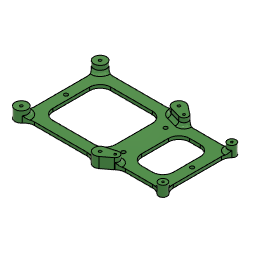
RFVplotter-PiAndMotorDriverMountingBracket-v1_0 (Autodesk Fusion 360 design; units mm, degrees)
Autodesk Fusion 360 part; units mm, degrees
sketch "Sketch1" plane through (0, 0, 0) normal (0, 1, 0) x (1, 0, 0)
  line L0 (72.5, 45) -> (-72.5, 45)
  line L1 (-72.5, 45) -> (-72.5, -45)
  line L2 (-72.5, -45) -> (72.5, -45)
  line L3 (72.5, -45) -> (72.5, 45)
  line L4 (72.5, 45) -> (-72.5, -45) construction
  line L5 (-72.5, 45) -> (72.5, -45) construction
  dimension "d1" = 90
  dimension "d2" = 145
  constraint horizontal L0
  constraint perpendicular L0 L1
  constraint parallel L0 L2
  constraint parallel L1 L3
  constraint coincident L4 origin
  constraint coincident L5 origin
  measures "d1" distance of L0.end L1.end
  measures "d2" distance of L1.end L2.end
extrude "Extrude1" add sketch "Sketch1" along normal blind 3 contours L0 L1 L2 L3 picked at (-24.166667, -15)
sketch "Sketch2" plane through (0, 3, 0) normal (0, 1, 0) x (-1, 0, 0)
  line L0 (-72.5, 45) -> (-72.5, -45)
  line L1 (-72.5, -45) -> (72.5, -45)
  line L2 (72.5, -45) -> (72.5, 45)
  line L3 (72.5, 45) -> (-72.5, 45)
  line L4 (65, -37.5) -> (-10, -37.5) construction
  line L5 (-10, -37.5) -> (-10, 37.5) construction
  line L6 (-10, 37.5) -> (65, 37.5) construction
  line L7 (65, 37.5) -> (65, -37.5) construction
  line L8 (65, -37.5) -> (-10, 37.5) construction
  line L9 (-10, -37.5) -> (65, 37.5) construction
  line L10 (0, 0) -> (72.5, 0) construction
  circle A0 centre (65, -37.5) radius 2.25 construction
  point P0 (27.5, 0)
  point P1 (65, 37.5)
  point P2 (-10, 37.5)
  point P3 (-10, -37.5)
  dimension "d5" = 75
  dimension "d6" = 75
  dimension "d7" = 4.5
  dimension "d8" = 7.5
  constraint horizontal L4
  constraint perpendicular L4 L5
  constraint parallel L4 L6
  constraint parallel L5 L7
  constraint coincident L8 P0
  constraint coincident L9 P0
  constraint midpoint L8 P0
  constraint coincident L10.start origin
  constraint midpoint L2 L10.end
  constraint coincident P0 L10
  constraint coincident L4.start L7.end
  constraint coincident P1 L6.end
  constraint coincident P2 L5.end
  constraint coincident P3 L4.end
  measures "d5" distance of L4 L6
  measures "d6" distance of P2 P1
  measures "d7" diameter of A0
  measures "d8" distance of L2 L7
hole "Hole1" at (-65, 3, 37.5) at (-65, 3, -37.5) at (10, 3, 37.5) at (10, 3, -37.5) direction (0, -1, 0) diameter 2.5 end through all
sketch "Sketch3" plane through (0, 3, 0) normal (0, 1, 0) x (-1, 0, 0)
  circle A0 centre (-10, 37.5) radius 1.25
  circle A1 centre (65, 37.5) radius 1.25
  circle A2 centre (65, -37.5) radius 1.25
  circle A3 centre (-10, -37.5) radius 1.25
  line L0 (-72.5, 45) -> (-72.5, -45)
  line L1 (-72.5, -45) -> (72.5, -45)
  line L2 (72.5, -45) -> (72.5, 45)
  line L3 (72.5, 45) -> (-72.5, 45)
  line L4 (-19.5, -32.75) -> (-65, -32.75) construction
  line L5 (-65, -32.75) -> (-65, 32.75) construction
  line L6 (-65, 32.75) -> (-19.5, 32.75) construction
  line L7 (-19.5, 32.75) -> (-19.5, -32.75) construction
  line L8 (-19.5, -32.75) -> (-65, 32.75) construction
  line L9 (-65, -32.75) -> (-19.5, 32.75) construction
  line L10 (0, 0) -> (-8.486168, 0)
  line L11 (-8.486168, 0) -> (-72.5, 0) construction
  point P0 (-42.25, 0)
  point P1 (-19.5, -32.75)
  point P2 (-65, -32.75)
  point P3 (-65, 32.75)
  point P4 (-19.5, 32.75)
  dimension "d12" = 65.5
  dimension "d13" = 45.5
  dimension "d14" = 7.5
  constraint horizontal L4
  constraint perpendicular L4 L5
  constraint parallel L4 L6
  constraint parallel L5 L7
  constraint coincident L8 P0
  constraint coincident L9 P0
  constraint coincident L10.start origin
  constraint perpendicular L7 L10
  constraint midpoint L0 L11.end
  constraint coincident P0 L11
  constraint coincident P1 L4.start
  constraint coincident P2 L4.end
  constraint coincident P3 L5.end
  constraint coincident P4 L6.end
  measures "d12" distance of P2 P3
  measures "d13" distance of P3 P4
  measures "d14" distance of L0 L5
hole "Hole2" at (19.5, 3, -32.75) at (65, 3, -32.75) at (65, 3, 32.75) at (19.5, 3, 32.75) direction (0, -1, 0) diameter 2 end through all
sketch "Sketch4" plane through (0, 3, 0) normal (0, 1, 0) x (-1, 0, 0)
  circle A0 centre (-65, 32.75) radius 1
  circle A1 centre (-19.5, -32.75) radius 1
  circle A2 centre (-65, -32.75) radius 1
  circle A3 centre (-19.5, 32.75) radius 1
  circle A4 centre (-10, 37.5) radius 1.25
  circle A5 centre (65, 37.5) radius 1.25
  circle A6 centre (65, -37.5) radius 1.25
  circle A7 centre (-10, -37.5) radius 1.25
  line L0 (-72.5, 45) -> (-72.5, -45)
  line L1 (-72.5, -45) -> (72.5, -45)
  line L2 (72.5, -45) -> (72.5, 45)
  line L3 (72.5, 45) -> (-72.5, 45)
  circle A8 centre (65, -37.5) radius 6
  circle A9 centre (65, 37.5) radius 6
  circle A10 centre (-10, -37.5) radius 6
  circle A11 centre (-10, 37.5) radius 6
  circle A12 centre (-19.5, -32.75) radius 4
  circle A13 centre (-65, -32.75) radius 4
  circle A14 centre (-19.5, 32.75) radius 4
  circle A15 centre (-65, 32.75) radius 4
  line L4 (65, -37.5) -> (-10, -37.5)
  line L5 (-10, -37.5) -> (-10, 37.5)
  line L6 (-10, 37.5) -> (65, 37.5)
  line L7 (65, 37.5) -> (65, -37.5)
  line L8 (65, -37.5) -> (-10, 37.5) construction
  line L9 (-10, -37.5) -> (65, 37.5) construction
  line L10 (-19.5, -32.75) -> (-65, -32.75)
  line L11 (-65, -32.75) -> (-65, 32.75)
  line L12 (-65, 32.75) -> (-19.5, 32.75)
  line L13 (-19.5, 32.75) -> (-19.5, -32.75)
  line L14 (-19.5, -32.75) -> (-65, 32.75) construction
  line L15 (-65, -32.75) -> (-19.5, 32.75) construction
  line L16 (-13.645808, -42.2653) -> (-21.930539, -35.926867)
  line L17 (-21.930539, 35.926867) -> (-13.645808, 42.2653)
  point P0 (27.5, 0)
  point P1 (-42.25, 0)
  dimension "d18" = 12
  dimension "d19" = 12
  dimension "d20" = 12
  dimension "d21" = 12
  dimension "d22" = 8
  dimension "d23" = 8
  dimension "d24" = 8
  dimension "d25" = 8
  constraint concentric A6 A8
  constraint concentric A5 A9
  constraint concentric A7 A10
  constraint concentric A4 A11
  constraint concentric A1 A12
  constraint concentric A2 A13
  constraint concentric A3 A14
  constraint concentric A0 A15
  constraint horizontal L4
  constraint perpendicular L4 L5
  constraint parallel L4 L6
  constraint parallel L5 L7
  constraint coincident L8 P0
  constraint coincident L9 P0
  constraint coincident A6.centre A8.centre
  constraint coincident A7.centre A10.centre
  constraint coincident A4.centre A11.centre
  constraint horizontal L10
  constraint perpendicular L10 L11
  constraint parallel L10 L12
  constraint parallel L11 L13
  constraint coincident L14 P1
  constraint coincident L15 P1
  constraint coincident A1.centre A12.centre
  constraint coincident A2.centre A13.centre
  constraint coincident A3.centre A14.centre
  constraint tangent A10 L16
  constraint tangent A12 L16
  constraint tangent A14 L17
  constraint tangent A11 L17
  measures "d18" diameter of A8
  measures "d19" diameter of A9
  measures "d20" diameter of A10
  measures "d21" diameter of A11
  measures "d22" diameter of A12
  measures "d23" diameter of A13
  measures "d24" diameter of A14
  measures "d25" diameter of A15
extrude "Extrude2" cut sketch "Sketch4" against normal through all contours L0 L1 L2 L3 picked at (-52.458043, -39.035927)
sketch "Sketch5" plane through (0, 3, 0) normal (0, 1, 0) x (-1, 0, 0)
  line L0 (-4, -37.5) -> (59, -37.5)
  arc A0 (59, -37.5) -> (65, -31.5) centre (65, -37.5) ccw
  line L1 (65, -31.5) -> (65, 31.5)
  arc A1 (65, 31.5) -> (59, 37.5) centre (65, 37.5) ccw
  line L2 (59, 37.5) -> (-4, 37.5)
  arc A2 (-4, 37.5) -> (-13.645808, 42.2653) centre (-10, 37.5) ccw
  line L3 (-13.645808, 42.2653) -> (-21.930539, 35.926867)
  arc A3 (-21.930539, 35.926867) -> (-23.5, 32.75) centre (-19.5, 32.75) ccw
  line L4 (-23.5, 32.75) -> (-61, 32.75)
  arc A4 (-61, 32.75) -> (-65, 28.75) centre (-65, 32.75) ccw
  line L5 (-65, 28.75) -> (-65, -28.75)
  arc A5 (-65, -28.75) -> (-61, -32.75) centre (-65, -32.75) ccw
  line L6 (-61, -32.75) -> (-23.5, -32.75)
  arc A6 (-23.5, -32.75) -> (-21.930539, -35.926867) centre (-19.5, -32.75) ccw
  line L7 (-21.930539, -35.926867) -> (-13.645808, -42.2653)
  arc A7 (-13.645808, -42.2653) -> (-4, -37.5) centre (-10, -37.5) ccw
  circle A8 centre (-65, 32.75) radius 1
  circle A9 centre (-19.5, -32.75) radius 1
  circle A10 centre (-65, -32.75) radius 1
  circle A11 centre (-19.5, 32.75) radius 1
  circle A12 centre (-10, 37.5) radius 1.25
  circle A13 centre (65, 37.5) radius 1.25
  circle A14 centre (65, -37.5) radius 1.25
  circle A15 centre (-10, -37.5) radius 1.25
  line L8 (-10, -37.5) -> (-10, 37.5) construction
  line L9 (-19.5, 32.75) -> (-19.5, -32.75) construction
  line L10 (-14.75, -41.420511) -> (-14.75, 41.420511) construction
  line L11 (0, 0) -> (-65, 0) construction
  point P0 (-14.75, -20)
  point P1 (-14.75, 20)
  dimension "d27" = 40
  constraint perpendicular L4 L8
  constraint coincident A7.centre A15.centre
  constraint coincident A2.centre A12.centre
  constraint coincident A3.centre A11.centre
  constraint coincident A6.centre A9.centre
  constraint parallel L9 L10
  constraint coincident L11.start origin
  constraint midpoint L5 L11.end
  constraint coincident L10 P0
  constraint coincident L10 P1
  constraint symmetric L11 P0 P1
  measures "d27" distance of P0 P1
hole "Hole3" at (14.75, 3, -20) at (14.75, 3, 20) direction (0, -1, 0) diameter 3.5 end through all
sketch "Sketch6" plane through (0, 3, 0) normal (0, 1, 0) x (-1, 0, 0)
  circle A0 centre (-14.75, -20) radius 1.75
  circle A1 centre (-14.75, 20) radius 1.75
  line L0 (-4, -37.5) -> (59, -37.5)
  arc A2 (59, -37.5) -> (65, -31.5) centre (65, -37.5) ccw
  line L1 (65, -31.5) -> (65, 31.5)
  arc A3 (65, 31.5) -> (59, 37.5) centre (65, 37.5) ccw
  line L2 (59, 37.5) -> (-4, 37.5)
  arc A4 (-4, 37.5) -> (-13.645808, 42.2653) centre (-10, 37.5) ccw
  line L3 (-13.645808, 42.2653) -> (-21.930539, 35.926867)
  arc A5 (-21.930539, 35.926867) -> (-23.5, 32.75) centre (-19.5, 32.75) ccw
  line L4 (-23.5, 32.75) -> (-61, 32.75)
  arc A6 (-61, 32.75) -> (-65, 28.75) centre (-65, 32.75) ccw
  line L5 (-65, 28.75) -> (-65, -28.75)
  arc A7 (-65, -28.75) -> (-61, -32.75) centre (-65, -32.75) ccw
  line L6 (-61, -32.75) -> (-23.5, -32.75)
  arc A8 (-23.5, -32.75) -> (-21.930539, -35.926867) centre (-19.5, -32.75) ccw
  line L7 (-21.930539, -35.926867) -> (-13.645808, -42.2653)
  arc A9 (-13.645808, -42.2653) -> (-4, -37.5) centre (-10, -37.5) ccw
  circle A10 centre (-65, 32.75) radius 1
  circle A11 centre (-19.5, -32.75) radius 1
  circle A12 centre (-65, -32.75) radius 1
  circle A13 centre (-19.5, 32.75) radius 1
  circle A14 centre (-10, 37.5) radius 1.25
  circle A15 centre (65, 37.5) radius 1.25
  circle A16 centre (65, -37.5) radius 1.25
  circle A17 centre (-10, -37.5) radius 1.25
  circle A18 centre (-19.5, 32.75) radius 4
  circle A19 centre (-19.5, -32.75) radius 4
  circle A20 centre (-65, 32.75) radius 4
  circle A21 centre (-65, -32.75) radius 4
  circle A22 centre (65, -37.5) radius 6
  circle A23 centre (65, 37.5) radius 6
  circle A24 centre (-10, 37.5) radius 6
  circle A25 centre (-10, -37.5) radius 6
  line L8 (-13.645808, -42.2653) -> (-21.930539, -35.926867)
  line L9 (-8.375245, -31.724174) -> (-18.41683, -28.899449)
  line L10 (0, 0) -> (-65, 0) construction
  line L11 (-8.375245, 31.724174) -> (-18.41683, 28.899449)
  line L12 (-13.645808, 42.2653) -> (-21.930539, 35.926867)
  constraint concentric A5 A18
  constraint concentric A8 A19
  constraint coincident L6.end A19
  constraint concentric A6 A20
  constraint coincident A6.end A20
  constraint concentric A7 A21
  constraint coincident A7.end A21
  constraint concentric A2 A22
  constraint coincident L0.end A22
  constraint concentric A3 A23
  constraint coincident A3.end A23
  constraint concentric A4 A24
  constraint coincident L2.end A24
  constraint concentric A9 A25
  constraint coincident L0.start A25
  constraint tangent A19 L8
  constraint tangent A25 L8
  constraint tangent A19 L9
  constraint tangent A25 L9
  constraint coincident L10.start origin
  constraint midpoint L5 L10.end
extrude "Extrude3" add sketch "Sketch6" along normal blind 7 contours A9 A25 | A2 A22 | L7 A19 A25 L8 L9 | A8 A19 | A3 A23 | A7 A21 | A4 A24 | L3 A18 A24 L11 L12 | A6 A20 | A5 A18 picked at (-12.390904, -41.1998) picked at (61.170181, -39.675192) picked at (-14.740196, -33.184319) picked at (-21.121713, -35.264646) picked at (60.605672, 37.798085) picked at (-65.220551, -29.765363) picked at (-12.390904, 41.1998) picked at (-14.740196, 33.184319) picked at (-65.220551, 29.765363) picked at (-21.121713, 35.264646)
sketch "Sketch7" plane through (0, 3, 0) normal (0, 1, 0) x (-1, 0, 0)
  arc A0 (-65, 28.75) -> (-61, 32.75) centre (-65, 32.75) ccw
  line L0 (-65, 28.75) -> (-65, -28.75)
  arc A1 (-61, -32.75) -> (-65, -28.75) centre (-65, -32.75) ccw
  line L1 (-61, -32.75) -> (-23.5, -32.75)
  arc A2 (-18.41683, -28.899449) -> (-23.5, -32.75) centre (-19.5, -32.75) ccw
  line L2 (-18.41683, -28.899449) -> (-8.375245, -31.724174)
  arc A3 (-4, -37.5) -> (-8.375245, -31.724174) centre (-10, -37.5) ccw
  line L3 (-4, -37.5) -> (59, -37.5)
  arc A4 (65, -31.5) -> (59, -37.5) centre (65, -37.5) ccw
  line L4 (65, -31.5) -> (65, 31.5)
  arc A5 (59, 37.5) -> (65, 31.5) centre (65, 37.5) ccw
  line L5 (59, 37.5) -> (-4, 37.5)
  arc A6 (-8.375245, 31.724174) -> (-4, 37.5) centre (-10, 37.5) ccw
  line L6 (-8.375245, 31.724174) -> (-18.41683, 28.899449)
  arc A7 (-23.5, 32.75) -> (-18.41683, 28.899449) centre (-19.5, 32.75) ccw
  line L7 (-23.5, 32.75) -> (-61, 32.75)
  circle A8 centre (-14.75, 20) radius 1.75
  circle A9 centre (-14.75, -20) radius 1.75
  line L8 (-4.75, 27.5) -> (55, 27.5)
  line L9 (55, 27.5) -> (55, -27.5)
  line L10 (55, -27.5) -> (-4.75, -27.5)
  line L11 (-4.75, -27.5) -> (-4.75, 27.5)
  line L12 (-4.75, 27.5) -> (55, -27.5) construction
  line L13 (55, 27.5) -> (-4.75, -27.5) construction
  line L14 (-55, 22.75) -> (-24.75, 22.75)
  line L15 (-24.75, 22.75) -> (-24.75, -22.75)
  line L16 (-24.75, -22.75) -> (-55, -22.75)
  line L17 (-55, -22.75) -> (-55, 22.75)
  line L18 (-55, 22.75) -> (-24.75, -22.75) construction
  line L19 (-24.75, 22.75) -> (-55, -22.75) construction
  line L20 (-65, 0) -> (65, 0) construction
  line L21 (-14.75, -20) -> (-14.75, 20) construction
  point P0 (25.125, 0)
  point P1 (-39.875, 0)
  dimension "d33" = 10
  dimension "d34" = 10
  dimension "d35" = 10
  dimension "d36" = 10
  dimension "d37" = 10
  dimension "d38" = 10
  constraint horizontal L8
  constraint perpendicular L8 L9
  constraint parallel L8 L10
  constraint parallel L9 L11
  constraint coincident L12 P0
  constraint coincident L13 P0
  constraint horizontal L14
  constraint perpendicular L14 L15
  constraint parallel L14 L16
  constraint parallel L15 L17
  constraint coincident L18 P1
  constraint coincident L19 P1
  constraint midpoint L0 L20.start
  constraint midpoint L4 L20.end
  constraint coincident P0 L20
  constraint coincident P1 L20
  constraint coincident A9.centre L21.start
  constraint coincident A8.centre L21.end
  measures "d33" distance of L4 L9
  measures "d34" distance of L3 L10
  measures "d35" distance of L1 L16
  measures "d36" distance of L0 L17
  measures "d37" distance of L15 L21
  measures "d38" distance of L11 L21
extrude "Extrude4" cut sketch "Sketch7" against normal through all contours L8 L9 L10 L11 | L14 L15 L16 L17 picked at (15.166667, 9.166667) picked at (-34.833333, 7.583333)
sketch "Sketch8" plane through (0, 3, 0) normal (0, 1, 0) x (-1, 0, 0)
  line L0 (-4.75, -27.5) -> (-4.75, 27.5)
  line L1 (-4.75, 27.5) -> (55, 27.5)
  line L2 (55, 27.5) -> (55, -27.5)
  line L3 (55, -27.5) -> (-4.75, -27.5)
  line L4 (-55, -22.75) -> (-55, 22.75)
  line L5 (-55, 22.75) -> (-24.75, 22.75)
  line L6 (-24.75, 22.75) -> (-24.75, -22.75)
  line L7 (-24.75, -22.75) -> (-55, -22.75)
  arc A0 (-65, 28.75) -> (-61, 32.75) centre (-65, 32.75) ccw
  line L8 (-65, 28.75) -> (-65, -28.75)
  arc A1 (-61, -32.75) -> (-65, -28.75) centre (-65, -32.75) ccw
  line L9 (-61, -32.75) -> (-23.5, -32.75)
  arc A2 (-18.41683, -28.899449) -> (-23.5, -32.75) centre (-19.5, -32.75) ccw
  line L10 (-18.41683, -28.899449) -> (-8.375245, -31.724174)
  arc A3 (-4, -37.5) -> (-8.375245, -31.724174) centre (-10, -37.5) ccw
  line L11 (-4, -37.5) -> (59, -37.5)
  arc A4 (65, -31.5) -> (59, -37.5) centre (65, -37.5) ccw
  line L12 (65, -31.5) -> (65, 31.5)
  arc A5 (59, 37.5) -> (65, 31.5) centre (65, 37.5) ccw
  line L13 (59, 37.5) -> (-4, 37.5)
  arc A6 (-8.375245, 31.724174) -> (-4, 37.5) centre (-10, 37.5) ccw
  line L14 (-8.375245, 31.724174) -> (-18.41683, 28.899449)
  arc A7 (-23.5, 32.75) -> (-18.41683, 28.899449) centre (-19.5, 32.75) ccw
  line L15 (-23.5, 32.75) -> (-61, 32.75)
  circle A8 centre (-14.75, 20) radius 1.75
  circle A9 centre (-14.75, -20) radius 1.75
  line L16 (-65, 0) -> (65, 0) construction
  point P0 (60, 0)
  point P1 (-60, 0)
  dimension "d48" = 5
  dimension "d49" = 5
  constraint midpoint L8 L16.start
  constraint midpoint L12 L16.end
  constraint coincident L16 P0
  constraint coincident L16 P1
  measures "d48" distance of L12 P0
  measures "d49" distance of L8 P1
hole "Hole4" at (-60, 3, 0) at (60, 3, 0) direction (0, -1, 0) diameter 3.5 end through all
fillet "Fillet1" radius 10 4 edges at (-55, 1.5, -27.5) (4.75, 1.5, -27.5) (4.75, 1.5, 27.5) (-55, 1.5, 27.5)
fillet "Fillet1" radius 10 4 edges at (24.75, 1.5, -22.75) (55, 1.5, -22.75) (55, 1.5, 22.75) (24.75, 1.5, 22.75)
fillet "Fillet2" radius 10 12 edges at (-65, 1.5, -31.5) (-59, 1.5, -37.5) (-65, 1.5, 31.5) (-59, 1.5, 37.5) (4, 1.5, 37.5) (23.5, 1.5, 32.75) (61, 1.5, 32.75) (65, 1.5, 28.75) (65, 1.5, -28.75) (61, 1.5, -32.75) (23.5, 1.5, -32.75) (4, 1.5, -37.5)
fillet "Fillet3" radius 3 10 edges at (-60.757359, 3, -33.257359) (-60.757359, 3, 33.257359) (22.961887, 3, -30.74617) (13.396037, 3, -30.311811) (4.287326, 3, -35.66551) (4.287326, 3, 35.66551) (13.396037, 3, 30.311811) (22.961887, 3, 30.74617) (62.171573, 3, 29.921573) (62.171573, 3, -29.921573)
equation "d12 = 68.5 mm - 3 mm"
equation "d13 = 48.5 mm - 3 mm"
equation "d19 = d18"
equation "d20 = d18"
equation "d21 = d18"
equation "d23 = d22"
equation "d24 = d22"
equation "d25 = d22"
equation "d49 = d48"
